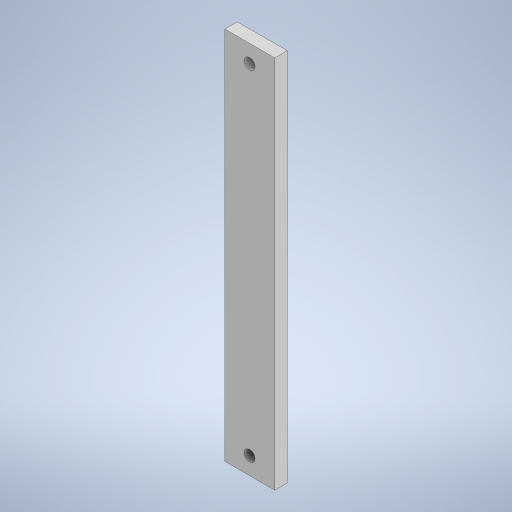
# Autodesk Inventor part: battery_plate
Saved by Autodesk Inventor 2023 (Build 270158000, 158)
## iProperties
Created: 2025-01-08
Part Number: battery_plate
Material: Všeobecné
Document SubType Name: Modeling
Designer: Marek
Density: 1 g/cm^3
Appearance: Výchozí
Author: Marek
## iProperties of the stored document battery_plate_3D tisk.ipt
Created: 2025-01-08
Part Number: battery_plate_3D tisk
Material: Všeobecné
Document SubType Name: Modeling
Designer: Marek
Density: 1 g/cm^3
Appearance: Výchozí
Author: Marek
Autodesk Inventor part; units mm, degrees
ref_plane "YZ Plane" through (0, 0, 0) normal (1, 0, 0) x (0, 1, 0)
ref_plane "XZ Plane" through (0, 0, 0) normal (0, 1, 0) x (-1, 0, 0)
ref_plane "XY Plane" through (0, 0, 0) normal (0, 0, 1) x (1, 0, 0)
sketch "Náčrt1" plane through (0, 0, 0) normal (0, 0, 1) x (1, 0, 0)
  line L0 (0, 52.5) -> (0, -52.5) projected
  line L1 (-7, 0) -> (7, 0) projected
  line L2 (-5, 37.5) -> (5, 37.5)
  line L3 (5, 37.5) -> (5, -37.5)
  line L4 (5, -37.5) -> (-5, -37.5)
  line L5 (-5, -37.5) -> (-5, 37.5)
  point P0 (0, 0)
  dimension "d0" = 75
  dimension "d1" = 10
  constraints: 8 end point, 2 parallel, 1 horizontal, 1 perpendicular, 2 other
  measures "d0" distance between parallel lines of L4 L2
  measures "d1" distance between parallel lines of L5 L3
extrude "Vysunutí1" add sketch "Náčrt1" along normal blind 2.5
sketch "Náčrt2" plane through (0, 0, 2.5) normal (0, 0, 1) x (1, 0, 0)
  line L0 (0, 52.5) -> (0, -52.5) projected
  line L1 (-7, 0) -> (7, 0) projected
  line L2 (-5, -37.5) -> (5, -37.5) projected
  line L3 (5, -37.5) -> (5, 37.5) projected
  line L4 (5, 37.5) -> (-5, 37.5) projected
  line L5 (-5, 37.5) -> (-5, -37.5) projected
  point P0 (0, 0)
  point P1 (0, 34)
  point P2 (0, -34)
  dimension "d4" = 3.5
  dimension "d5" = 3.5
  constraints: 2 point on line
  measures "d4" distance from line of L4 point (0, 34)
  measures "d5" distance from line of L2 point (0, -34)
hole "Díra1" at (0, 34, 2.5) at (0, -34, 2.5) direction (0, 0, -1) diameter 2.15 end through all
